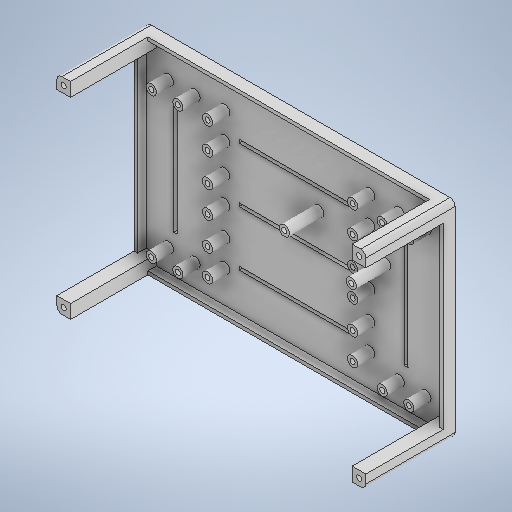
# Autodesk Inventor part: reduced_tortoise
Saved by Autodesk Inventor 2025.1 (Build 291241000, 241)
## iProperties
Created: 2025-04-09
Part Number: reduced_tortoise
Material: Generic
Document SubType Name: Modeling
Designer: Ian Ching
Density: 1 g/cm^3
Appearance: Default
Author: Ian Ching
Autodesk Inventor part; units mm, degrees
ref_plane "YZ Plane" through (0, 0, 0) normal (1, 0, 0) x (0, 1, 0)
ref_plane "XZ Plane" through (0, 0, 0) normal (0, 1, 0) x (-1, 0, 0)
ref_plane "XY Plane" through (0, 0, 0) normal (0, 0, 1) x (1, 0, 0)
sketch "Sketch2" plane through (0, 0, 0) normal (0, 0, 1) x (1, 0, 0)
  line L0 (0, 0) -> (180, 0)
  line L1 (180, 0) -> (180, -120)
  line L2 (180, -120) -> (0, -120)
  line L3 (0, -120) -> (0, 0)
  dimension "d0" = 180
  dimension "d1" = 120
  constraints: 8 end point, 2 parallel, 1 coincident, 1 horizontal, 1 perpendicular
  measures "d0" distance of L1.end L2.end
  measures "d1" distance of L0.end L1.end
extrude "Extrusion1" add sketch "Sketch2" along normal blind 2
sketch "Sketch3" plane through (0, 0, 2) normal (0, 0, 1) x (1, 0, 0)
  line L0 (15, -20.5) -> (30.5, -20.5)
  line L1 (30.5, -20.5) -> (30.5, -105)
  line L2 (30.5, -105) -> (15, -105)
  line L3 (15, -105) -> (15, -20.5)
  line L4 (18, -29) -> (20, -29)
  line L5 (20, -29) -> (20, -96)
  line L6 (20, -96) -> (18, -96)
  line L7 (18, -96) -> (18, -29)
  line L8 (15, -105) -> (18, -105)
  line L9 (18, -105) -> (18, -96)
  line L10 (18, -96) -> (15, -96)
  line L11 (15, -96) -> (15, -105)
  circle A0 centre (15, -20.5) radius 1.5
  circle A1 centre (30.5, -20.5) radius 1.5
  circle A2 centre (15, -105) radius 1.5
  circle A3 centre (30.5, -105) radius 1.5
  line L12 (149.5, -20.5) -> (165, -20.5)
  line L13 (165, -20.5) -> (165, -105)
  line L14 (165, -105) -> (149.5, -105)
  line L15 (149.5, -105) -> (149.5, -20.5)
  line L16 (152.5, -29) -> (154.5, -29)
  line L17 (154.5, -29) -> (154.5, -96)
  line L18 (154.5, -96) -> (152.5, -96)
  line L19 (152.5, -96) -> (152.5, -29)
  line L20 (149.5, -105) -> (152.5, -105)
  line L21 (152.5, -105) -> (152.5, -96)
  line L22 (152.5, -96) -> (149.5, -96)
  line L23 (149.5, -96) -> (149.5, -105)
  circle A4 centre (149.5, -20.5) radius 1.5
  circle A5 centre (165, -20.5) radius 1.5
  circle A6 centre (149.5, -105) radius 1.5
  line L24 (47.75, -99) -> (47.75, -83.5)
  line L25 (47.75, -83.5) -> (132.25, -83.5)
  line L26 (132.25, -83.5) -> (132.25, -99)
  line L27 (132.25, -99) -> (47.75, -99)
  circle A7 centre (47.75, -99) radius 1.5
  circle A8 centre (47.75, -83.5) radius 1.5
  circle A9 centre (132.25, -99) radius 1.5
  circle A10 centre (132.25, -83.5) radius 1.5
  line L28 (0, -120) -> (180, -120) projected
  line L29 (180, 0) -> (0, 0) projected
  line L30 (90, 0) -> (90, -120)
  line L31 (0, 0) -> (0, -120) projected
  line L32 (90, -120) -> (47.75, -120)
  line L33 (47.75, -120) -> (47.75, -99)
  line L34 (47.75, -99) -> (90, -99)
  line L35 (90, -99) -> (90, -120)
  line L36 (132.25, -99) -> (123.25, -99)
  line L37 (123.25, -99) -> (123.25, -96)
  line L38 (123.25, -96) -> (132.25, -96)
  line L39 (132.25, -96) -> (132.25, -99)
  line L40 (123.25, -96) -> (56.25, -96)
  line L41 (56.25, -96) -> (56.25, -94)
  line L42 (56.25, -94) -> (123.25, -94)
  line L43 (123.25, -94) -> (123.25, -96)
  circle A11 centre (15, -20.5) radius 3
  circle A12 centre (30.5, -20.5) radius 3
  circle A13 centre (15, -105) radius 3
  circle A14 centre (30.5, -105) radius 3
  circle A15 centre (149.5, -105) radius 3
  circle A16 centre (165, -105) radius 3
  circle A17 centre (149.5, -20.5) radius 3
  circle A18 centre (165, -20.5) radius 3
  circle A19 centre (47.75, -83.5) radius 3
  circle A20 centre (47.75, -99) radius 3
  circle A21 centre (132.25, -83.5) radius 3
  circle A22 centre (132.25, -99) radius 3
  circle A23 centre (47.75, -51.5) radius 1.5
  circle A24 centre (47.75, -51.5) radius 3
  circle A25 centre (47.75, -67) radius 1.5
  circle A26 centre (47.75, -67) radius 3
  line L44 (132.25, -67) -> (47.75, -67)
  line L45 (47.75, -67) -> (47.75, -51.5)
  line L46 (47.75, -51.5) -> (132.25, -51.5)
  line L47 (56.25, -62) -> (123.25, -62)
  line L48 (123.25, -64) -> (56.25, -64)
  line L49 (56.25, -64) -> (56.25, -62)
  line L50 (47.75, -67) -> (90, -67)
  line L51 (123.25, -67) -> (123.25, -64)
  line L52 (123.25, -62) -> (123.25, -64)
  line L53 (132.25, -67) -> (123.25, -67)
  line L54 (123.25, -64) -> (132.25, -64)
  line L55 (132.25, -64) -> (132.25, -67)
  circle A27 centre (132.25, -67) radius 1.5
  circle A28 centre (132.25, -67) radius 3
  line L56 (132.25, -51.5) -> (132.25, -67)
  circle A29 centre (132.25, -51.5) radius 1.5
  circle A30 centre (132.25, -51.5) radius 3
  circle A31 centre (47.75, -19.5) radius 1.5
  circle A32 centre (47.75, -19.5) radius 3
  circle A33 centre (47.75, -35) radius 1.5
  circle A34 centre (47.75, -35) radius 3
  line L57 (132.25, -35) -> (47.75, -35)
  line L58 (47.75, -35) -> (47.75, -19.5)
  line L59 (47.75, -19.5) -> (132.25, -19.5)
  line L60 (56.25, -30) -> (123.25, -30)
  line L61 (123.25, -32) -> (56.25, -32)
  line L62 (56.25, -32) -> (56.25, -30)
  line L63 (47.75, -35) -> (90, -35)
  line L64 (123.25, -35) -> (123.25, -32)
  line L65 (123.25, -30) -> (123.25, -32)
  line L66 (132.25, -35) -> (123.25, -35)
  line L67 (123.25, -32) -> (132.25, -32)
  line L68 (132.25, -32) -> (132.25, -35)
  circle A35 centre (132.25, -35) radius 1.5
  circle A36 centre (132.25, -35) radius 3
  line L69 (132.25, -19.5) -> (132.25, -35)
  circle A37 centre (132.25, -19.5) radius 1.5
  circle A38 centre (132.25, -19.5) radius 3
  line L70 (0, -120) -> (15, -120)
  line L71 (15, -120) -> (15, -105)
  line L72 (15, -105) -> (0, -105)
  line L73 (0, -105) -> (0, -120)
  line L74 (180, -120) -> (165, -120)
  line L75 (165, -120) -> (165, -105)
  line L76 (165, -105) -> (180, -105)
  line L77 (180, -105) -> (180, -120)
  circle A39 centre (165, -105) radius 1.5
  point P0 (90, -99)
  point P1 (83.5338, -99)
  point P2 (90, -67)
  point P3 (83.5338, -67)
  point P4 (90, -35)
  point P5 (83.5338, -35)
  point P6 (90, -30)
  point P7 (90, -32)
  point P8 (90, -94)
  point P9 (90, -96)
  dimension "d4" = 15.5
  dimension "d5" = 84.5
  dimension "d6" = 2
  dimension "d7" = 67
  dimension "d10" = 3
  dimension "d11" = 9
  dimension "d12" = 3
  dimension "d13" = 3
  dimension "d14" = 3
  dimension "d15" = 3
  dimension "d16" = 15.5
  dimension "d17" = 84.5
  dimension "d18" = 2
  dimension "d19" = 67
  dimension "d20" = 3
  dimension "d21" = 9
  dimension "d22" = 3
  dimension "d23" = 3
  dimension "d24" = 3
  dimension "d26" = 15.5
  dimension "d27" = 84.5
  dimension "d32" = 3
  dimension "d33" = 3
  dimension "d34" = 3
  dimension "d35" = 3
  dimension "d96" = 42.25
  dimension "d97" = 21
  dimension "d98" = 9
  dimension "d99" = 3
  dimension "d100" = 67
  dimension "d101" = 2
  dimension "d131" = 6
  dimension "d132" = 6
  dimension "d133" = 6
  dimension "d134" = 6
  dimension "d135" = 6
  dimension "d136" = 6
  dimension "d137" = 6
  dimension "d138" = 6
  dimension "d139" = 6
  dimension "d140" = 6
  dimension "d141" = 6
  dimension "d142" = 6
  dimension "d145" = 32
  dimension "d150" = 15
  dimension "d151" = 15
  dimension "d152" = 15
  dimension "d153" = 15
  dimension "d154" = 3
  constraints: 150 end point, 43 coincident, 40 centre point, 24 parallel, 12 perpendicular, 11 horizontal, 4 point on line, 3 midpoint, 1 vertical, 86 other
  measures "d4" distance of L2.end L1.end
  measures "d5" distance of L0.end L1.end
  measures "d6" distance of L6.end L5.end
  measures "d7" distance of L4.end L5.end
  measures "d10" distance of L10.end L6.end
  measures "d11" distance of L6.end L8.end
  measures "d12" diameter of A0
  measures "d13" diameter of A1
  measures "d14" diameter of A2
  measures "d15" diameter of A3
  measures "d16" distance of L14.start L15.start
  measures "d17" distance of L14.start L12.end
  measures "d18" distance of L19.start L17.end
  measures "d19" distance of L17.start L17.end
  measures "d20" distance of L22.end L19.start
  measures "d21" distance of L19.start L21.start
  measures "d22" diameter of A4
  measures "d23" diameter of A5
  measures "d24" diameter of A6
  measures "d26" distance of L26.start L27.start
  measures "d27" distance of L24.end L26.start
  measures "d32" diameter of A7
  measures "d33" diameter of A8
  measures "d34" diameter of A9
  measures "d35" diameter of A10
  measures "d96" distance of L33.end L34.end
  measures "d97" distance of L32.end L33.end
  measures "d98" distance of L37.end L38.end
  measures "d99" distance of L36.end L37.end
  measures "d100" distance of L41.end L42.end
  measures "d101" distance of L40.end L41.end
  measures "d131" diameter of A11
  measures "d132" diameter of A12
  measures "d133" diameter of A13
  measures "d134" diameter of A14
  measures "d135" diameter of A15
  measures "d136" diameter of A16
  measures "d137" diameter of A17
  measures "d138" diameter of A18
  measures "d139" diameter of A19
  measures "d140" diameter of A20
  measures "d141" diameter of A21
  measures "d142" diameter of A22
  measures "d145" distance of A20.centre A26.centre
  measures "d150" distance of L72.end L2.end
  measures "d151" distance of L2.end L70.end
  measures "d152" distance of L14.start L76.end
  measures "d153" distance of L74.end L14.start
  measures "d154" diameter of A39
sketch "Sketch4" plane through (0, 0, 2) normal (0, 0, 1) x (1, 0, 0)
  line L0 (180, 0) -> (0, 0) projected
  line L1 (0, 0) -> (8, 0)
  line L2 (8, 0) -> (8, -8)
  line L3 (8, -8) -> (0, -8)
  line L4 (0, -8) -> (0, 0)
  line L5 (90, 0) -> (90, -120)
  line L6 (0, -120) -> (180, -120) projected
  line L7 (0, 0) -> (0, -120) projected
  line L8 (0, -60) -> (180, -60)
  line L9 (180, -120) -> (180, 0) projected
  line L10 (180, 0) -> (172, 0)
  line L11 (172, 0) -> (172, -8)
  line L12 (172, -8) -> (180, -8)
  line L13 (180, -8) -> (180, 0)
  line L14 (0, -120) -> (8, -120)
  line L15 (8, -120) -> (8, -112)
  line L16 (8, -112) -> (0, -112)
  line L17 (0, -112) -> (0, -120)
  line L18 (180, -120) -> (172, -120)
  line L19 (172, -120) -> (172, -112)
  line L20 (172, -112) -> (180, -112)
  line L21 (180, -112) -> (180, -120)
  point P0 (172, 0)
  point P1 (180, -112)
  point P2 (172, -120)
  point P3 (0, -112)
  point P4 (8, -120)
  point P5 (8, 0)
  dimension "d56" = 8
  dimension "d57" = 8
  constraints: 36 end point, 9 symmetric about line, 4 midpoint, 2 parallel, 1 horizontal, 1 perpendicular
  measures "d56" distance of L2.end L3.end
  measures "d57" distance of L1.end L2.end
extrude "Extrusion2" add sketch "Sketch3" along normal blind 10 contours L3 A0 L0 | L0 A0 L3 | A0 L3 A11 L0 | L0 A11 L3 A0 | A12 L1 A1 L0 | L0 A1 L1 A12 | A1 L1 L0 | L0 L1 A1 | A13 L2 A2 L3 | L3 A2 L72 A13 | A14 L2 A3 L1 | L1 A3 L2 A14 | A2 L2 L3 | L3 L72 A2 | A13 L71 A2 L2 | L72 A2 L71 A13 | A3 L2 L1 | L1 L2 A3 | L2 A2 L71 | L71 A2 L72 | A20 L24 A7 L33 | L33 A7 L27 A20 | L33 L27 A7 | A7 L24 L33 | A20 L27 A7 L24 | L59 A31 L58 A32 | A32 L58 A31 L59 | A38 L69 A37 L59 | L59 A37 L69 A38 | L75 A39 L76 A16 | A16 L14 A39 L75 | A7 L27 L24 | A19 L25 A8 L24 | L24 A8 L25 A19 | L59 L58 A31 | A31 L58 L59 | A37 L69 L59 | L59 L69 A37 | A16 L13 A39 L14 | L76 A39 L13 A16 | A39 L14 L75 | L75 L76 A39 | A22 L26 A9 L27 | L27 A9 L26 A22 | A8 L25 L24 | L24 L25 A8 | L58 A33 L57 A34 | A34 L57 A33 L58 | A36 L57 A35 L68 | L68 A35 L57 A36 | A39 L13 L14 | A15 L15 A6 L14 | L14 A6 L15 A15 | L76 L13 A39 | A9 L26 L27 | L27 L26 A9 | L58 L57 A33 | A33 L57 L58 | A35 L57 L68 | L68 L57 A35 | A6 L15 L14 | L14 L15 A6 | A18 L12 A5 L13 | L13 A5 L12 A18 | A21 L25 A10 L26 | L26 A10 L25 A21 | L46 A23 L45 A24 | A24 L45 A23 L46 | A30 L56 A29 L46 | L46 A29 L56 A30 | A5 L12 L13 | L13 L12 A5 | A10 L25 L26 | L26 L25 A10 | L44 A25 L45 A26 | A26 L45 A25 L44 | L46 L45 A23 | A23 L45 L46 | A29 L56 L46 | L46 L56 A29 | A17 L12 A4 L15 | L15 A4 L12 A17 | A28 L55 A27 L44 | L44 A27 L55 A28 | L44 L45 A25 | A25 L45 L44 | A4 L12 L15 | L15 L12 A4 | A27 L55 L44 | L44 L55 A27
sketch "Sketch6" plane through (0, 0, 2) normal (0, 0, 1) x (1, 0, 0)
  line L0 (100, -58) -> (154, -58)
  line L1 (154, -58) -> (154, -20)
  line L2 (154, -20) -> (100, -20)
  line L3 (100, -20) -> (100, -58)
  line L4 (0, -120) -> (180, -120) projected
  line L5 (100, -58) -> (102.5, -58)
  line L6 (102.5, -58) -> (102.5, -43)
  line L7 (102.5, -43) -> (100, -43)
  line L8 (100, -43) -> (100, -58)
  line L9 (154, -58) -> (141.5, -58)
  line L10 (141.5, -58) -> (141.5, -50)
  line L11 (141.5, -50) -> (154, -50)
  line L12 (154, -50) -> (154, -58)
  circle A0 centre (102.5, -43) radius 1.5
  circle A1 centre (102.5, -43) radius 3
  circle A2 centre (141.5, -50) radius 1.5
  circle A3 centre (141.5, -50) radius 3
  line L13 (0, -120) -> (180, -120) projected
  line L14 (180, -120) -> (154, -120)
  line L15 (154, -120) -> (154, -58)
  line L16 (154, -58) -> (180, -58)
  line L17 (180, -58) -> (180, -120)
  point P0 (0, 0)
  dimension "d115" = 54
  dimension "d116" = 38
  dimension "d209" = 2.5
  dimension "d210" = 15
  dimension "d211" = 12.5
  dimension "d212" = 8
  dimension "d213" = 3
  dimension "d214" = 6
  dimension "d215" = 3
  dimension "d216" = 6
  dimension "d217" = 26
  dimension "d218" = 62
  constraints: 32 end point, 8 parallel, 4 centre point, 4 coincident, 4 horizontal, 4 perpendicular
  measures "d115" distance of L2.end L1.end
  measures "d116" distance of L0.end L1.end
  measures "d209" distance of L7.end L6.end
  measures "d210" distance of L6.end L5.end
  measures "d211" distance of L10.end L11.end
  measures "d212" distance of L9.end L10.end
  measures "d213" diameter of A0
  measures "d214" diameter of A1
  measures "d215" diameter of A2
  measures "d216" diameter of A3
  measures "d217" distance of L0.end L16.end
  measures "d218" distance of L14.end L0.end
sketch "Sketch7" plane through (15, -20.5, 12) normal (0, 0, 1) x (1, 0, 0)
  circle A0 centre (0, 0) radius 3 projected
  circle A1 centre (0, 0) radius 1.5
  circle A2 centre (15.5, 0) radius 3 projected
  circle A3 centre (15.5, 0) radius 1.5
  circle A4 centre (32.75, 1) radius 3 projected
  circle A5 centre (32.75, 1) radius 1.5
  circle A6 centre (32.75, -14.5) radius 3 projected
  circle A7 centre (32.75, -14.5) radius 1.5
  circle A8 centre (117.25, 1) radius 3 projected
  circle A9 centre (117.25, 1) radius 1.5
  circle A10 centre (117.25, -14.5) radius 3 projected
  circle A11 centre (117.25, -14.5) radius 1.5
  circle A12 centre (134.5, 0) radius 3 projected
  circle A13 centre (134.5, 0) radius 1.5
  circle A14 centre (150, 0) radius 3 projected
  circle A15 centre (150, 0) radius 1.5
  circle A16 centre (134.5, -84.5) radius 3 projected
  circle A17 centre (134.5, -84.5) radius 1.5
  circle A18 centre (150, -84.5) radius 3 projected
  circle A19 centre (150, -84.5) radius 1.5
  circle A20 centre (117.25, -31) radius 3 projected
  circle A21 centre (117.25, -31) radius 1.5
  circle A22 centre (117.25, -46.5) radius 3 projected
  circle A23 centre (117.25, -46.5) radius 1.5
  circle A24 centre (117.25, -63) radius 3 projected
  circle A25 centre (117.25, -63) radius 1.5
  circle A26 centre (117.25, -78.5) radius 3 projected
  circle A27 centre (117.25, -78.5) radius 1.5
  circle A28 centre (32.75, -31) radius 3 projected
  circle A29 centre (32.75, -31) radius 1.5
  circle A30 centre (32.75, -46.5) radius 3 projected
  circle A31 centre (32.75, -46.5) radius 1.5
  circle A32 centre (32.75, -63) radius 3 projected
  circle A33 centre (32.75, -63) radius 1.5
  circle A34 centre (32.75, -78.5) radius 3 projected
  circle A35 centre (32.75, -78.5) radius 1.5
  circle A36 centre (0, -84.5) radius 3 projected
  circle A37 centre (0, -84.5) radius 1.5
  circle A38 centre (15.5, -84.5) radius 3 projected
  circle A39 centre (15.5, -84.5) radius 1.5
  line L0 (3, -8.5) -> (5, -8.5) projected
  line L1 (5, -8.5) -> (5, -75.5) projected
  line L2 (3, -8.5) -> (5, -8.5)
  line L3 (5, -8.5) -> (5, -75.5)
  line L4 (5, -75.5) -> (3, -75.5)
  line L5 (3, -75.5) -> (3, -8.5)
  line L6 (118.25, -73.5) -> (118.25, -75.5) projected
  line L7 (118.25, -73.5) -> (85, -73.5) projected
  line L8 (118.25, -75.5) -> (51.25, -75.5)
  line L9 (51.25, -75.5) -> (51.25, -73.5)
  line L10 (51.25, -73.5) -> (118.25, -73.5)
  line L11 (118.25, -73.5) -> (118.25, -75.5)
  line L12 (51.25, -41.5) -> (51.25, -43.5) projected
  line L13 (51.25, -43.5) -> (118.25, -43.5) projected
  line L14 (51.25, -41.5) -> (118.25, -41.5)
  line L15 (118.25, -41.5) -> (118.25, -43.5)
  line L16 (118.25, -43.5) -> (51.25, -43.5)
  line L17 (51.25, -43.5) -> (51.25, -41.5)
  line L18 (118.25, -9.5) -> (85, -9.5) projected
  line L19 (85, -11.5) -> (118.25, -11.5) projected
  line L20 (51.25, -9.5) -> (118.25, -9.5)
  line L21 (118.25, -9.5) -> (118.25, -11.5)
  line L22 (118.25, -11.5) -> (51.25, -11.5)
  line L23 (51.25, -11.5) -> (51.25, -9.5)
  line L24 (157.5, -75.5) -> (157.5, -8.5) projected
  line L25 (159.5, -75.5) -> (159.5, -8.5) projected
  line L26 (157.5, -8.5) -> (159.5, -8.5)
  line L27 (159.5, -8.5) -> (159.5, -75.5)
  line L28 (159.5, -75.5) -> (157.5, -75.5)
  line L29 (157.5, -75.5) -> (157.5, -8.5)
  point P0 (-15, 20.5)
  point P1 (51.25, -11.5)
  dimension "d157" = 3
  dimension "d158" = 3
  dimension "d159" = 3
  dimension "d160" = 3
  dimension "d161" = 3
  dimension "d162" = 3
  dimension "d163" = 3
  dimension "d164" = 3
  dimension "d165" = 3
  dimension "d166" = 3
  dimension "d167" = 3
  dimension "d168" = 3
  dimension "d169" = 3
  dimension "d170" = 3
  dimension "d171" = 3
  dimension "d172" = 3
  dimension "d173" = 3
  dimension "d174" = 3
  dimension "d175" = 3
  dimension "d176" = 3
  constraints: 40 end point, 20 centre point, 20 coincident, 10 parallel, 5 horizontal, 5 perpendicular
  measures "d157" diameter of A1
  measures "d158" diameter of A3
  measures "d159" diameter of A5
  measures "d160" diameter of A7
  measures "d161" diameter of A9
  measures "d162" diameter of A11
  measures "d163" diameter of A13
  measures "d164" diameter of A15
  measures "d165" diameter of A17
  measures "d166" diameter of A19
  measures "d167" diameter of A21
  measures "d168" diameter of A23
  measures "d169" diameter of A25
  measures "d170" diameter of A27
  measures "d171" diameter of A29
  measures "d172" diameter of A31
  measures "d173" diameter of A33
  measures "d174" diameter of A35
  measures "d175" diameter of A37
  measures "d176" diameter of A39
extrude "Extrusion3" cut sketch "Sketch7" against normal blind 10 contours A1 | A3 | A5 | A7 | A9 | A11 | A13 | A15 | A17 | A19 | A21 | A23 | A25 | A27 | A29 | A31 | A33 | A35 | A37 | A39
sketch "Sketch9" plane through (0, 0, 2) normal (0, 0, 1) x (1, 0, 0)
  line L0 (0, 0) -> (0, -120) projected
  line L1 (0, -120) -> (15, -120)
  line L2 (15, -120) -> (15, -105)
  line L3 (15, -105) -> (0, -105)
  line L4 (0, -105) -> (0, -120)
  circle A0 centre (15, -105) radius 3 projected
  circle A1 centre (30.5, -20.5) radius 1.5 projected
  line L5 (15, -105) -> (30.5, -105)
  line L6 (30.5, -105) -> (30.5, -20.5)
  line L7 (30.5, -20.5) -> (15, -20.5)
  line L8 (15, -20.5) -> (15, -105)
  line L9 (15, -105) -> (18, -105)
  line L10 (18, -105) -> (18, -96)
  line L11 (18, -96) -> (15, -96)
  line L12 (15, -96) -> (15, -105)
  line L13 (18, -96) -> (20, -96)
  line L14 (20, -96) -> (20, -29)
  line L15 (20, -29) -> (18, -29)
  line L16 (18, -29) -> (18, -96)
  circle A2 centre (165, -105) radius 3 projected
  line L17 (180, -120) -> (165, -120)
  line L18 (165, -120) -> (165, -105)
  line L19 (165, -105) -> (180, -105)
  line L20 (180, -105) -> (180, -120)
  line L21 (165, -105) -> (149.5, -105)
  line L22 (149.5, -105) -> (149.5, -20.5)
  line L23 (149.5, -20.5) -> (165, -20.5)
  line L24 (165, -20.5) -> (165, -105)
  circle A3 centre (149.5, -105) radius 1.5 projected
  line L25 (149.5, -105) -> (152.5, -105)
  line L26 (152.5, -105) -> (152.5, -96)
  line L27 (152.5, -96) -> (149.5, -96)
  line L28 (149.5, -96) -> (149.5, -105)
  line L29 (152.5, -96) -> (154.5, -96)
  line L30 (154.5, -96) -> (154.5, -29)
  line L31 (154.5, -29) -> (152.5, -29)
  line L32 (152.5, -29) -> (152.5, -96)
  circle A4 centre (132.25, -99) radius 1.5 projected
  circle A5 centre (47.75, -83.5) radius 1.5 projected
  line L33 (132.25, -99) -> (47.75, -99)
  line L34 (47.75, -99) -> (47.75, -83.5)
  line L35 (47.75, -83.5) -> (132.25, -83.5)
  line L36 (132.25, -83.5) -> (132.25, -99)
  line L37 (132.25, -99) -> (123.25, -99)
  line L38 (123.25, -99) -> (123.25, -96)
  line L39 (123.25, -96) -> (132.25, -96)
  line L40 (132.25, -96) -> (132.25, -99)
  line L41 (123.25, -96) -> (56.25, -96)
  line L42 (56.25, -96) -> (56.25, -94)
  line L43 (56.25, -94) -> (123.25, -94)
  line L44 (123.25, -94) -> (123.25, -96)
  circle A6 centre (132.25, -67) radius 1.5 projected
  circle A7 centre (47.75, -51.5) radius 1.5 projected
  line L45 (132.25, -67) -> (47.75, -67)
  line L46 (47.75, -67) -> (47.75, -51.5)
  line L47 (47.75, -51.5) -> (132.25, -51.5)
  line L48 (132.25, -51.5) -> (132.25, -67)
  line L49 (132.25, -67) -> (123.25, -67)
  line L50 (123.25, -67) -> (123.25, -64)
  line L51 (123.25, -64) -> (132.25, -64)
  line L52 (132.25, -64) -> (132.25, -67)
  line L53 (123.25, -64) -> (56.25, -64)
  line L54 (56.25, -64) -> (56.25, -62)
  line L55 (56.25, -62) -> (123.25, -62)
  line L56 (123.25, -62) -> (123.25, -64)
  circle A8 centre (132.25, -35) radius 1.5 projected
  circle A9 centre (47.75, -19.5) radius 1.5 projected
  line L57 (132.25, -35) -> (47.75, -35)
  line L58 (47.75, -35) -> (47.75, -19.5)
  line L59 (47.75, -19.5) -> (132.25, -19.5)
  line L60 (132.25, -19.5) -> (132.25, -35)
  circle A10 centre (132.25, -35) radius 3 projected
  line L61 (132.25, -35) -> (123.25, -35)
  line L62 (123.25, -35) -> (123.25, -32)
  line L63 (123.25, -32) -> (132.25, -32)
  line L64 (132.25, -32) -> (132.25, -35)
  line L65 (123.25, -32) -> (56.25, -32)
  line L66 (56.25, -32) -> (56.25, -30)
  line L67 (56.25, -30) -> (123.25, -30)
  line L68 (123.25, -30) -> (123.25, -32)
  dimension "d179" = 15
  dimension "d180" = 15
  dimension "d181" = 15.5
  dimension "d182" = 84.5
  dimension "d183" = 3
  dimension "d184" = 9
  dimension "d185" = 2
  dimension "d186" = 67
  dimension "d187" = 15
  dimension "d188" = 15
  dimension "d189" = 15.5
  dimension "d190" = 84.5
  dimension "d191" = 3
  dimension "d192" = 9
  dimension "d193" = 2
  dimension "d194" = 67
  dimension "d195" = 9
  dimension "d196" = 3
  dimension "d197" = 67
  dimension "d198" = 2
  dimension "d199" = 9
  dimension "d200" = 3
  dimension "d201" = 67
  dimension "d202" = 2
  dimension "d203" = 9
  dimension "d204" = 3
  dimension "d205" = 67
  dimension "d206" = 2
  constraints: 136 end point, 34 parallel, 17 horizontal, 17 perpendicular
  measures "d179" distance of L3.end L2.end
  measures "d180" distance of L2.end L1.end
  measures "d181" distance of L7.end L6.end
  measures "d182" distance of L6.end L5.end
  measures "d183" distance of L11.end L10.end
  measures "d184" distance of L10.end L9.end
  measures "d185" distance of L15.end L14.end
  measures "d186" distance of L14.end L13.end
  measures "d187" distance of L18.end L19.end
  measures "d188" distance of L17.end L18.end
  measures "d189" distance of L22.end L23.end
  measures "d190" distance of L21.end L22.end
  measures "d191" distance of L27.end L26.end
  measures "d192" distance of L26.end L25.end
  measures "d193" distance of L31.end L30.end
  measures "d194" distance of L30.end L29.end
  measures "d195" distance of L38.end L39.end
  measures "d196" distance of L37.end L38.end
  measures "d197" distance of L42.end L43.end
  measures "d198" distance of L41.end L42.end
  measures "d199" distance of L50.end L51.end
  measures "d200" distance of L49.end L50.end
  measures "d201" distance of L54.end L55.end
  measures "d202" distance of L53.end L54.end
  measures "d203" distance of L62.end L63.end
  measures "d204" distance of L61.end L62.end
  measures "d205" distance of L66.end L67.end
  measures "d206" distance of L65.end L66.end
extrude "Extrusion4" cut sketch "Sketch9" against normal blind 10 contours L16 L15 L14 L13 | L32 L31 L30 L29 | L41 L42 L43 L44 | L53 L54 L55 L56 | L65 L66 L67 L68
extrude "Extrusion5" add sketch "Sketch6" along normal blind 20 contours A1 L3 | L3 L7 A0 L6 A1 | L6 A0 L7 L3 A1 | A3 L11 A2 L10 | L10 A2 L11 A3 | A0 L7 L6 | L6 L7 A0 | A2 L11 L10 | L10 L11 A2
sketch "Sketch10" plane through (102.5, -43, 22) normal (0, 0, 1) x (1, 0, 0)
  circle A0 centre (0, 0) radius 3 projected
  circle A1 centre (0, 0) radius 1.5
  circle A2 centre (39, -7) radius 3 projected
  circle A3 centre (39, -7) radius 1.5
  point P0 (-102.5, 43)
  point P1 (36.7167, -8.9459)
  point P2 (36.0333, -6.5541)
  dimension "d221" = 3
  dimension "d222" = 3
  constraints: 2 centre point, 2 coincident
  measures "d221" diameter of A1
  measures "d222" diameter of A3
extrude "Extrusion6" cut sketch "Sketch10" against normal blind 10 contours A1 | A3
sketch "Sketch12" plane through (0, 0, 2) normal (0, 0, 1) x (1, 0, 0)
  line L0 (0, -120) -> (180, -120) projected
  line L1 (180, 0) -> (0, 0) projected
  line L2 (0, -120) -> (2, -120)
  line L3 (2, -120) -> (2, 0)
  line L4 (2, 0) -> (0, 0)
  line L5 (0, 0) -> (0, -120)
  line L6 (180, -120) -> (180, 0) projected
  line L7 (0, -120) -> (180, -120)
  line L8 (180, -120) -> (180, -118)
  line L9 (180, -118) -> (0, -118)
  line L10 (0, -118) -> (0, -120)
  line L11 (180, 0) -> (178, 0)
  line L12 (178, 0) -> (178, -120)
  line L13 (178, -120) -> (180, -120)
  line L14 (180, -120) -> (180, 0)
  line L15 (180, 0) -> (0, 0)
  line L16 (0, 0) -> (0, -2)
  line L17 (0, -2) -> (180, -2)
  line L18 (180, -2) -> (180, 0)
  point P0 (2, -118)
  point P1 (2, -2)
  point P2 (178, -2)
  point P3 (178, -118)
  dimension "d225" = 2
  dimension "d226" = 2
  dimension "d227" = 2
  dimension "d228" = 2
  constraints: 32 end point, 8 parallel, 4 horizontal, 4 perpendicular, 4 point on line
  measures "d225" distance of L4.end L3.end
  measures "d226" distance of L8.end L7.end
  measures "d227" distance of L13.end L12.end
  measures "d228" distance of L16.end L15.end
extrude "Extrusion7" add sketch "Sketch12" along normal blind 5 contours L5 L9 L3 L0 | L3 L9 L12 L0 | L5 L17 L3 L9 | L12 L9 L6 L0 | L5 L1 L3 L17 | L12 L17 L6 L9 | L3 L1 L12 L17 | L12 L1 L6 L17
extrude "Extrusion8" add sketch "Sketch4" along normal blind 50 contours L9 L12 L11 L0 | L2 L3 L4 L0 | L9 L6 L19 L20 | L6 L7 L16 L15
fillet "Fillet1" radius 3 4 edges at (0, -120, 26) (180, -120, 26) (180, 0, 26) (0, 0, 26)
sketch "Sketch13" plane through (0, 0, 52) normal (0, 0, 1) x (1, 0, 0)
  line L0 (0, 0) -> (4, 0)
  line L1 (4, 0) -> (4, -4)
  line L2 (4, -4) -> (0, -4)
  line L3 (0, -4) -> (0, 0)
  circle A0 centre (4, -4) radius 1.5
  line L4 (177, 0) -> (3, 0) projected
  line L5 (90, 0) -> (90, -120)
  line L6 (8, -120) -> (172, -120) projected
  line L7 (0, -8) -> (0, -112) projected
  line L8 (0, -60) -> (180, -60)
  line L9 (180, -117) -> (180, -3) projected
  circle A1 centre (176, -4) radius 1.5
  circle A2 centre (4, -116) radius 1.5
  circle A3 centre (176, -116) radius 1.5
  dimension "d234" = 4
  dimension "d235" = 4
  dimension "d236" = 3
  constraints: 12 end point, 4 centre point, 4 midpoint, 3 symmetric about line, 2 parallel, 1 coincident, 1 horizontal, 1 perpendicular, 3 other
  measures "d234" distance of L1.end L2.end
  measures "d235" distance of L0.end L1.end
  measures "d236" diameter of A0
extrude "Extrusion9" cut sketch "Sketch13" against normal blind 10 contours A0 L1 L2 | L2 L1 A0 | A1 | A2 | A3
body "Solid1"
